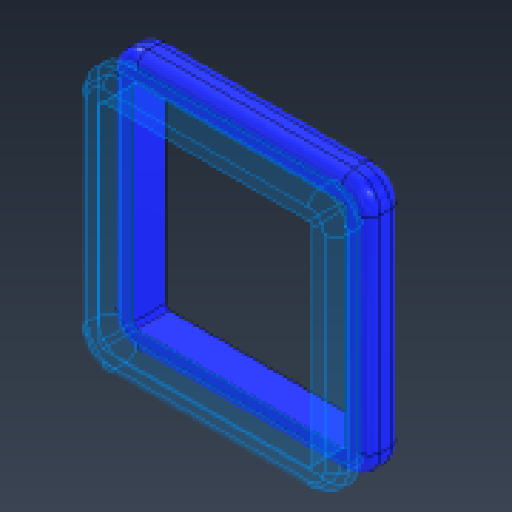
# Autodesk Inventor part: Bumpers
Saved by Autodesk Inventor 2026 (Build 300175050, 175E)
## iProperties
Created: 2026-01-21
Part Number: Bumpers
Material: Spruce
Document SubType Name: Modeling
Designer: Jthib
Mass: 9348.75 g
Surface Area: 10216.2 cm^2
Volume: 23371.9 cm^3
Density: 0.4 g/cm^3
Appearance: Blue - Wall Paint - Glossy
Author: Jthib
Autodesk Inventor part; units mm, degrees
ref_plane "YZ Plane" through (0, 0, 0) normal (1, 0, 0) x (0, 1, 0)
ref_plane "XZ Plane" through (0, 0, 0) normal (0, 1, 0) x (-1, 0, 0)
ref_plane "XY Plane" through (0, 0, 0) normal (0, 0, 1) x (1, 0, 0)
sketch "Sketch1" plane through (0, 0, 0) normal (0, 0, 1) x (1, 0, 0)
  line L0 (-349.25, 0) -> (-349.25, 336.55)
  line L1 (-336.55, 349.25) -> (336.55, 349.25)
  line L2 (349.25, 336.55) -> (349.25, -336.55)
  line L3 (336.55, -349.25) -> (-336.55, -349.25)
  line L4 (-349.25, -336.55) -> (-349.25, 0)
  arc A0 (-336.55, 349.25) -> (-349.25, 336.55) centre (-336.55, 336.55) ccw
  arc A1 (349.25, 336.55) -> (336.55, 349.25) centre (336.55, 336.55) ccw
  arc A2 (336.55, -349.25) -> (349.25, -336.55) centre (336.55, -336.55) ccw
  arc A3 (-349.25, -336.55) -> (-336.55, -349.25) centre (-336.55, -336.55) ccw
  point P0 (0, 0)
  point P1 (-349.25, 349.25)
  point P2 (349.25, 349.25)
  point P3 (349.25, -349.25)
  point P4 (-349.25, -349.25)
  dimension "d0" = 698.5
  dimension "d1" = 698.5
  dimension "d2" = 349.25
  dimension "d3" = 349.25
  dimension "d9" = 12.7
  constraints: 10 end point, 9 point on line, 8 point on circle, 8 tangent, 4 centre point, 4 perpendicular, 3 equal radius, 1 collinear, 1 vertical
  measures "d0" distance of point (349.25, 349.25) point (349.25, -349.25)
  measures "d1" distance of point (-349.25, 349.25) point (349.25, 349.25)
  measures "d2" distance from line of point (0, 0) L1
  measures "d3" distance from line of L2 point (0, 0)
  measures "d9" radius of A0
sketch "Sketch2" plane through (0, 0, 0) normal (0, 1, 0) x (-1, 0, 0)
  line L0 (393.7, 53.975) -> (349.25, 53.975)
  line L1 (349.25, 53.975) -> (349.25, -53.975)
  line L2 (349.25, -53.975) -> (393.7, -53.975)
  line L3 (425.45, -22.225) -> (425.45, 22.225)
  arc A0 (425.45, 22.225) -> (393.7, 53.975) centre (393.7, 22.225) ccw
  arc A1 (393.7, -53.975) -> (425.45, -22.225) centre (393.7, -22.225) ccw
  point P0 (0, 0)
  point P1 (425.45, 53.975)
  point P2 (349.25, 0)
  point P3 (349.25, 0)
  point P4 (349.25, 0)
  point P5 (349.25, 0)
  dimension "d4" = 107.95
  dimension "d5" = 76.2
  dimension "d6" = 31.75
  constraints: 8 end point, 4 point on circle, 4 tangent, 2 centre point, 2 parallel, 2 point on line, 1 coincident, 1 equal radius, 1 horizontal, 1 midpoint, 1 perpendicular
  measures "d4" distance of L0.end L1.end
  measures "d5" distance of point (425.45, 53.975) L0.end
  measures "d6" radius of A0
sweep "Sweep1" add profiles "Sketch2" path "Sketch1" path curves L0 A0 L1 A1 L2 A2 L3 A3 L4
sketch "Sketch3" plane through (425.45, -336.55, 22.225) normal (1, 0, 0) x (0, 0, -1)
  line L0 (-22.225, 82.55) -> (-22.225, 590.55) construction
  line L1 (-22.225, 590.55) -> (66.675, 590.55) construction
  line L2 (66.675, 590.55) -> (66.675, 82.55) construction
  line L3 (66.675, 82.55) -> (-22.225, 82.55) construction
  line L4 (-22.225, 82.55) -> (66.675, 590.55) construction
  spline S0 degree 2 poles (60.325, 210.0554) (60.325, 204.3206) (56.3041, 199.3768) (52.0195, 199.3768) knots 0 0 0 1 2 2 2
  spline S1 degree 2 poles (52.0195, 199.3768) (50.1738, 199.3768) (47.4053, 199.9701) knots 0 0 0 1 1 1
  line L5 (47.4053, 199.9701) -> (35.5402, 202.409)
  line L6 (35.5402, 202.409) -> (35.5402, 218.1632)
  line L7 (35.5402, 218.1632) -> (42.4615, 216.713)
  spline S2 degree 2 poles (42.4615, 216.713) (42.9888, 216.5811) (43.9117, 216.4493) (44.3731, 216.4493) knots 0 0 0 1 2 2 2
  spline S3 degree 2 poles (44.3731, 216.4493) (45.4937, 216.4493) (46.2847, 217.7017) (46.2847, 219.4156) knots 0 0 0 1 2 2 2
  line L8 (46.2847, 219.4156) -> (46.2847, 240.7727)
  spline S4 degree 2 poles (46.2847, 240.7727) (46.2847, 243.3434) (44.7027, 245.0573) (42.4615, 245.6505) knots 0 0 0 1 2 2 2
  line L9 (42.4615, 245.6505) -> (29.7395, 248.3531)
  spline S5 degree 2 poles (29.7395, 248.3531) (29.1463, 248.419) (28.3553, 248.5509) (28.0257, 248.5509) knots 0 0 0 1 2 2 2
  spline S6 degree 2 poles (28.0257, 248.5509) (25.9823, 248.5509) (25.9823, 245.6505) knots 0 0 0 1 1 1
  line L10 (25.9823, 245.6505) -> (25.9823, 204.4524)
  line L11 (25.9823, 204.4524) -> (-15.875, 213.3512)
  line L12 (-15.875, 213.3512) -> (-15.875, 271.9514)
  line L13 (-15.875, 271.9514) -> (-1.3074, 268.9192)
  line L14 (-1.3074, 268.9192) -> (-1.3074, 226.4028)
  line L15 (-1.3074, 226.4028) -> (13.3921, 223.2388)
  line L16 (13.3921, 223.2388) -> (13.3921, 257.186)
  spline S7 degree 2 poles (13.3921, 257.186) (13.3921, 261.8002) (17.3471, 266.0189) (20.9726, 266.0189) knots 0 0 0 1 2 2 2
  spline S8 degree 2 poles (20.9726, 266.0189) (22.4887, 266.0189) (24.2025, 265.6234) knots 0 0 0 1 1 1
  line L17 (24.2025, 265.6234) -> (47.0757, 260.8114)
  spline S9 degree 2 poles (47.0757, 260.8114) (53.7992, 259.3612) (60.325, 252.374) (60.325, 245.0573) knots 0 0 0 1 2 2 2
  line L18 (60.325, 245.0573) -> (60.325, 210.0554)
  spline S10 degree 2 poles (60.325, 282.7618) (60.325, 277.027) (56.3041, 271.9514) (52.0195, 271.9514) knots 0 0 0 1 2 2 2
  spline S11 degree 2 poles (52.0195, 271.9514) (50.1738, 271.9514) (47.4053, 272.5446) knots 0 0 0 1 1 1
  line L19 (47.4053, 272.5446) -> (29.2781, 276.3678)
  spline S12 degree 2 poles (29.2781, 276.3678) (24.9935, 277.2907) (21.3022, 283.2232) (20.9726, 287.1782) knots 0 0 0 1 2 2 2
  spline S13 degree 2 poles (20.9726, 287.1782) (20.5771, 283.8824) (17.5449, 280.3228) (14.315, 280.3228) knots 0 0 0 1 2 2 2
  spline S14 degree 2 poles (14.315, 280.3228) (13.0625, 280.3228) (11.3487, 280.6524) knots 0 0 0 1 1 1
  line L20 (11.3487, 280.6524) -> (-2.8894, 283.6846)
  spline S15 degree 2 poles (-2.8894, 283.6846) (-9.4151, 285.0689) (-15.875, 292.5834) (-15.875, 299.7683) knots 0 0 0 1 2 2 2
  line L21 (-15.875, 299.7683) -> (-15.875, 332.9905)
  spline S16 degree 2 poles (-15.875, 332.9905) (-15.875, 338.923) (-11.5904, 344.1304) (-7.3058, 344.1304) knots 0 0 0 1 2 2 2
  spline S17 degree 2 poles (-7.3058, 344.1304) (-5.0646, 344.1304) (-2.8894, 343.669) knots 0 0 0 1 1 1
  line L22 (-2.8894, 343.669) -> (11.3487, 340.6369)
  spline S18 degree 2 poles (11.3487, 340.6369) (16.0947, 339.5822) (20.5112, 334.1111) (20.9726, 330.0242) knots 0 0 0 1 2 2 2
  spline S19 degree 2 poles (20.9726, 330.0242) (21.3022, 333.3201) (24.0048, 337.4728) (27.0369, 337.4728) knots 0 0 0 1 2 2 2
  spline S20 degree 2 poles (27.0369, 337.4728) (27.5643, 337.4728) (28.6849, 337.341) (29.2781, 337.2751) knots 0 0 0 1 2 2 2
  line L23 (29.2781, 337.2751) -> (47.4053, 333.4519)
  spline S21 degree 2 poles (47.4053, 333.4519) (53.9311, 332.0676) (60.325, 325.0804) (60.325, 317.7637) knots 0 0 0 1 2 2 2
  line L24 (60.325, 317.7637) -> (60.325, 282.7618)
  spline S22 degree 2 poles (30.201, 321.3891) (29.7395, 321.5209) (28.9485, 321.5209) knots 0 0 0 1 1 1
  spline S23 degree 2 poles (28.9485, 321.5209) (27.6961, 321.5209) (26.7733, 320.0048) (26.7733, 318.0933) knots 0 0 0 1 2 2 2
  line L25 (26.7733, 318.0933) -> (26.7733, 296.6043)
  spline S24 degree 2 poles (26.7733, 296.6043) (26.7733, 294.3631) (28.2234, 292.122) (30.201, 291.7924) knots 0 0 0 1 2 2 2
  line L26 (30.201, 291.7924) -> (42.1978, 289.2875)
  spline S25 degree 2 poles (42.1978, 289.2875) (42.7911, 289.2216) (43.5821, 289.0898) (43.9117, 289.0898) knots 0 0 0 1 2 2 2
  spline S26 degree 2 poles (43.9117, 289.0898) (46.2847, 289.0898) (46.2847, 292.4516) knots 0 0 0 1 1 1
  line L27 (46.2847, 292.4516) -> (46.2847, 313.9405)
  spline S27 degree 2 poles (46.2847, 313.9405) (46.2847, 316.1817) (44.439, 318.4228) (42.1978, 318.8843) knots 0 0 0 1 2 2 2
  line L28 (42.1978, 318.8843) -> (30.201, 321.3891)
  spline S28 degree 2 poles (1.7248, 327.2557) (1.1316, 327.3216) (0.4724, 327.4535) (0.1428, 327.4535) knots 0 0 0 1 2 2 2
  spline S29 degree 2 poles (0.1428, 327.4535) (-2.0984, 327.4535) (-2.0984, 324.0917) knots 0 0 0 1 1 1
  line L29 (-2.0984, 324.0917) -> (-2.0984, 302.8005)
  spline S30 degree 2 poles (-2.0984, 302.8005) (-2.0984, 300.5593) (-0.5163, 298.5159) (1.7248, 298.1204) knots 0 0 0 1 2 2 2
  line L30 (1.7248, 298.1204) -> (12.5352, 295.8133)
  spline S31 degree 2 poles (12.5352, 295.8133) (12.9307, 295.7474) (13.6558, 295.6156) (13.9854, 295.6156) knots 0 0 0 1 2 2 2
  spline S32 degree 2 poles (13.9854, 295.6156) (15.9629, 295.6156) (15.9629, 298.8455) knots 0 0 0 1 1 1
  line L31 (15.9629, 298.8455) -> (15.9629, 320.4003)
  spline S33 degree 2 poles (15.9629, 320.4003) (15.9629, 322.6415) (14.4468, 324.5531) (12.5352, 324.9486) knots 0 0 0 1 2 2 2
  line L32 (12.5352, 324.9486) -> (1.7248, 327.2557)
  spline S34 degree 2 poles (60.325, 355.2045) (60.325, 349.4697) (56.3041, 344.3941) (52.0195, 344.3941) knots 0 0 0 1 2 2 2
  spline S35 degree 2 poles (52.0195, 344.3941) (50.1738, 344.3941) (47.4053, 344.9874) knots 0 0 0 1 1 1
  line L33 (47.4053, 344.9874) -> (29.2781, 348.8106)
  spline S36 degree 2 poles (29.2781, 348.8106) (24.9935, 349.7334) (21.3022, 355.6659) (20.9726, 359.6209) knots 0 0 0 1 2 2 2
  spline S37 degree 2 poles (20.9726, 359.6209) (20.5771, 356.3251) (17.5449, 352.7656) (14.315, 352.7656) knots 0 0 0 1 2 2 2
  spline S38 degree 2 poles (14.315, 352.7656) (13.0625, 352.7656) (11.3487, 353.0952) knots 0 0 0 1 1 1
  line L34 (11.3487, 353.0952) -> (-2.8894, 356.1273)
  spline S39 degree 2 poles (-2.8894, 356.1273) (-9.4151, 357.5116) (-15.875, 365.0261) (-15.875, 372.2111) knots 0 0 0 1 2 2 2
  line L35 (-15.875, 372.2111) -> (-15.875, 405.4332)
  spline S40 degree 2 poles (-15.875, 405.4332) (-15.875, 411.3657) (-11.5904, 416.5732) (-7.3058, 416.5732) knots 0 0 0 1 2 2 2
  spline S41 degree 2 poles (-7.3058, 416.5732) (-5.0646, 416.5732) (-2.8894, 416.1118) knots 0 0 0 1 1 1
  line L36 (-2.8894, 416.1118) -> (11.3487, 413.0796)
  spline S42 degree 2 poles (11.3487, 413.0796) (16.0947, 412.0249) (20.5112, 406.5538) (20.9726, 402.467) knots 0 0 0 1 2 2 2
  spline S43 degree 2 poles (20.9726, 402.467) (21.3022, 405.7628) (24.0048, 409.9156) (27.0369, 409.9156) knots 0 0 0 1 2 2 2
  spline S44 degree 2 poles (27.0369, 409.9156) (27.5643, 409.9156) (28.6849, 409.7837) (29.2781, 409.7178) knots 0 0 0 1 2 2 2
  line L37 (29.2781, 409.7178) -> (47.4053, 405.8946)
  spline S45 degree 2 poles (47.4053, 405.8946) (53.9311, 404.5104) (60.325, 397.5232) (60.325, 390.2064) knots 0 0 0 1 2 2 2
  line L38 (60.325, 390.2064) -> (60.325, 355.2045)
  spline S46 degree 2 poles (30.201, 393.8318) (29.7395, 393.9637) (28.9485, 393.9637) knots 0 0 0 1 1 1
  spline S47 degree 2 poles (28.9485, 393.9637) (27.6961, 393.9637) (26.7733, 392.4476) (26.7733, 390.536) knots 0 0 0 1 2 2 2
  line L39 (26.7733, 390.536) -> (26.7733, 369.0471)
  spline S48 degree 2 poles (26.7733, 369.0471) (26.7733, 366.8059) (28.2234, 364.5647) (30.201, 364.2351) knots 0 0 0 1 2 2 2
  line L40 (30.201, 364.2351) -> (42.1978, 361.7303)
  spline S49 degree 2 poles (42.1978, 361.7303) (42.7911, 361.6644) (43.5821, 361.5325) (43.9117, 361.5325) knots 0 0 0 1 2 2 2
  spline S50 degree 2 poles (43.9117, 361.5325) (46.2847, 361.5325) (46.2847, 364.8943) knots 0 0 0 1 1 1
  line L41 (46.2847, 364.8943) -> (46.2847, 386.3832)
  spline S51 degree 2 poles (46.2847, 386.3832) (46.2847, 388.6244) (44.439, 390.8656) (42.1978, 391.327) knots 0 0 0 1 2 2 2
  line L42 (42.1978, 391.327) -> (30.201, 393.8318)
  spline S52 degree 2 poles (1.7248, 399.6984) (1.1316, 399.7644) (0.4724, 399.8962) (0.1428, 399.8962) knots 0 0 0 1 2 2 2
  spline S53 degree 2 poles (0.1428, 399.8962) (-2.0984, 399.8962) (-2.0984, 396.5344) knots 0 0 0 1 1 1
  line L43 (-2.0984, 396.5344) -> (-2.0984, 375.2433)
  spline S54 degree 2 poles (-2.0984, 375.2433) (-2.0984, 373.0021) (-0.5163, 370.9586) (1.7248, 370.5631) knots 0 0 0 1 2 2 2
  line L44 (1.7248, 370.5631) -> (12.5352, 368.2561)
  spline S55 degree 2 poles (12.5352, 368.2561) (12.9307, 368.1901) (13.6558, 368.0583) (13.9854, 368.0583) knots 0 0 0 1 2 2 2
  spline S56 degree 2 poles (13.9854, 368.0583) (15.9629, 368.0583) (15.9629, 371.2882) knots 0 0 0 1 1 1
  line L45 (15.9629, 371.2882) -> (15.9629, 392.8431)
  spline S57 degree 2 poles (15.9629, 392.8431) (15.9629, 395.0843) (14.4468, 396.9958) (12.5352, 397.3913) knots 0 0 0 1 2 2 2
  line L46 (12.5352, 397.3913) -> (1.7248, 399.6984)
  spline S58 degree 2 poles (60.325, 428.1086) (60.325, 422.3739) (56.3041, 417.4301) (52.0195, 417.4301) knots 0 0 0 1 2 2 2
  spline S59 degree 2 poles (52.0195, 417.4301) (50.1738, 417.4301) (47.4053, 418.0234) knots 0 0 0 1 1 1
  line L47 (47.4053, 418.0234) -> (35.5402, 420.4623)
  line L48 (35.5402, 420.4623) -> (35.5402, 436.2164)
  line L49 (35.5402, 436.2164) -> (42.4615, 434.7663)
  spline S60 degree 2 poles (42.4615, 434.7663) (42.9888, 434.6344) (43.9117, 434.5026) (44.3731, 434.5026) knots 0 0 0 1 2 2 2
  spline S61 degree 2 poles (44.3731, 434.5026) (45.4937, 434.5026) (46.2847, 435.755) (46.2847, 437.4689) knots 0 0 0 1 2 2 2
  line L50 (46.2847, 437.4689) -> (46.2847, 458.8259)
  spline S62 degree 2 poles (46.2847, 458.8259) (46.2847, 461.3967) (44.7027, 463.1106) (42.4615, 463.7038) knots 0 0 0 1 2 2 2
  line L51 (42.4615, 463.7038) -> (29.7395, 466.4064)
  spline S63 degree 2 poles (29.7395, 466.4064) (29.1463, 466.4723) (28.3553, 466.6041) (28.0257, 466.6041) knots 0 0 0 1 2 2 2
  spline S64 degree 2 poles (28.0257, 466.6041) (25.9823, 466.6041) (25.9823, 463.7038) knots 0 0 0 1 1 1
  line L52 (25.9823, 463.7038) -> (25.9823, 422.5057)
  line L53 (25.9823, 422.5057) -> (-15.875, 431.4045)
  line L54 (-15.875, 431.4045) -> (-15.875, 490.0047)
  line L55 (-15.875, 490.0047) -> (-1.3074, 486.9725)
  line L56 (-1.3074, 486.9725) -> (-1.3074, 444.4561)
  line L57 (-1.3074, 444.4561) -> (13.3921, 441.292)
  line L58 (13.3921, 441.292) -> (13.3921, 475.2393)
  spline S65 degree 2 poles (13.3921, 475.2393) (13.3921, 479.8535) (17.3471, 484.0721) (20.9726, 484.0721) knots 0 0 0 1 2 2 2
  spline S66 degree 2 poles (20.9726, 484.0721) (22.4887, 484.0721) (24.2025, 483.6766) knots 0 0 0 1 1 1
  line L59 (24.2025, 483.6766) -> (47.0757, 478.8647)
  spline S67 degree 2 poles (47.0757, 478.8647) (53.7992, 477.4145) (60.325, 470.4273) (60.325, 463.1106) knots 0 0 0 1 2 2 2
  line L60 (60.325, 463.1106) -> (60.325, 428.1086)
  point P0 (22.225, 336.55)
  point P1 (22.225, 336.55)
  dimension "d2" = 349.25
  dimension "d10" = 508
  dimension "d11" = 88.9
  constraints: 2 end point, 1 coincident, 1 horizontal, 1 midpoint, 2 other
  measures "d10" distance of L0.start L0.end
  measures "d11" distance of L0.end L1.end
emboss "Emboss1" sketch "Sketch3" operation cut depth 0.254 direction (-1, 0, 0)
pattern_circular "Circular Pattern1" count 4 over 360 about axis through (0, 0, -10) along (0, 0, 1) of "Emboss1"
equation "\"d0\" = d1"
equation "\"d2\" = 0.5 * d0"
equation "\"d3\" = 0.5 * d1"
body "Solid1"
